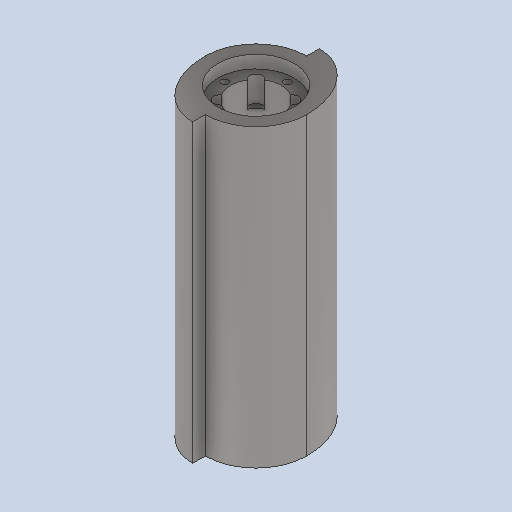
# Autodesk Inventor part: Деталь1
Saved by Autodesk Inventor 2024.2 (Build 282272000, 272)
## iProperties
Created: 2025-03-01
Part Number: Деталь1
Material: Сталь, литейная
Document SubType Name: Modeling
Designer: Timofey
Density: 7.85 g/cm^3
Appearance: С умеренной полировкой
Author: Timofey
Autodesk Inventor part; units mm, degrees
ref_plane "YZ Plane" through (0, 0, 0) normal (1, 0, 0) x (0, 1, 0)
ref_plane "XZ Plane" through (0, 0, 0) normal (0, 1, 0) x (-1, 0, 0)
ref_plane "XY Plane" through (0, 0, 0) normal (0, 0, 1) x (1, 0, 0)
sketch "Эскиз1" plane through (0, 0, 0) normal (0, 1, 0) x (-1, 0, 0)
  line L0 (0, 60) -> (0, 75)
  line L1 (0, -60) -> (0, -75)
  ellipse E0 centre (0, 0) end of major axis (0, -75) minor radius 60 (60, 0) -> (0, 75) ccw
  ellipse E1 centre (0, 0) end of major axis (0, -75) minor radius 60 (-60, 0) -> (0, -75) ccw
  arc A0 (0, 60) -> (-60, 0) centre (0, 0) ccw
  arc A1 (0, -60) -> (60, 0) centre (0, 0) ccw
  circle A2 centre (0, 0) radius 30
  dimension "d1" = 75
  dimension "d2" = 75
  dimension "d5" = 60
  constraints: 5 point on circle, 4 end point, 4 vertical, 3 centre point, 3 coincident, 9 other
  measures "d1" distance of A0.centre L0.end
  measures "d2" distance of A0.centre L1.end
  measures "d5" diameter of A2
extrude "Выдавливание1" add sketch "Эскиз1" along normal blind 350 contours L0 E0 A1 L1 E1 A0 | A2
sketch "Эскиз2" plane through (0, 0, 0) normal (0, -1, 0) x (1, 0, 0)
  ellipse E0 centre (0, 0) end of major axis (0, -75) minor radius 60 (0, 75) -> (-60, 0) ccw projected
  line L0 (0, 75) -> (0, 0)
  circle A0 centre (0, 0) radius 30
  line L1 (0, -75) -> (0, -60) projected
  line L2 (0, 0) -> (0, -75)
  line L3 (0, 0) -> (26.5165, -26.5165)
  line L4 (0, 0) -> (37.5, 0) construction
  line L5 (0, 0) -> (-26.5165, -26.5165)
  line L6 (0, 0) -> (37.5, 0) construction
  line L7 (0, 0) -> (-26.5165, 26.5165)
  line L8 (0, 0) -> (37.5, 0) construction
  line L9 (0, 0) -> (26.5165, 26.5165)
  line L10 (0, 0) -> (37.5, 0) construction
  circle A1 centre (26.5165, 26.5165) radius 5
  circle A2 centre (26.5165, -26.5165) radius 5
  circle A3 centre (-26.5165, 26.5165) radius 5
  circle A4 centre (-26.5165, -26.5165) radius 5
  circle A5 centre (0, 0) radius 45
  line L11 (0, 0) -> (30, 0)
  circle A6 centre (30, 0) radius 5
  line L12 (0, 0) -> (0, -30)
  circle A7 centre (0, -30) radius 5
  line L13 (0, 0) -> (-30, 0)
  circle A8 centre (-30, 0) radius 5
  line L14 (0, 0) -> (0, 30)
  circle A9 centre (0, 30) radius 5
  dimension "d13" = 60
  dimension "d14" = 37.5
  dimension "d15" = 45
  dimension "d16" = 37.5
  dimension "d17" = 135
  dimension "d18" = 37.5
  dimension "d19" = 135
  dimension "d20" = 37.5
  dimension "d21" = 45
  dimension "d22" = 10
  dimension "d23" = 10
  dimension "d24" = 10
  dimension "d25" = 10
  dimension "d26" = 90
  dimension "d30" = 30
  dimension "d31" = 30
  dimension "d32" = 30
  dimension "d33" = 30
  constraints: 28 end point, 10 centre point, 10 coincident, 5 horizontal, 4 equal length, 3 point on line, 1 collinear, 1 perpendicular, 1 vertical, 1 other
  measures "d13" diameter of A0
  measures "d14" distance of L2.start L3.end
  measures "d15" angle of L3 L4
  measures "d16" distance of L2.start L5.end
  measures "d17" angle of L5 L6
  measures "d18" distance of L2.start L7.end
  measures "d19" angle of L8 L7
  measures "d20" distance of L2.start L9.end
  measures "d21" angle of L10 L9
  measures "d22" diameter of A1
  measures "d23" diameter of A2
  measures "d24" diameter of A3
  measures "d25" diameter of A4
  measures "d26" diameter of A5
  measures "d30" distance of L11.start L11.end
  measures "d31" distance of L11.start L12.end
  measures "d32" distance of L11.start L13.end
  measures "d33" distance of L11.start L14.end
hole "Отверстие1" at (0, 0, 0) direction (0, 1, 0) diameter 60 end through all counterbore diameter 90 counterbore depth 15
sketch "Эскиз3" plane through (0, 0, 0) normal (0, -1, 0) x (1, 0, 0)
  line L0 (0, 0) -> (30, 0)
  circle A0 centre (30, 0) radius 5
  line L1 (0, 0) -> (0, -30)
  circle A1 centre (0, 0) radius 30 projected
  circle A2 centre (0, -30) radius 5
  line L2 (0, 0) -> (-30, 0)
  line L3 (0, 0) -> (0, 30)
  circle A3 centre (0, 30) radius 5
  circle A4 centre (-30, 0) radius 5
  dimension "d34" = 30
  dimension "d35" = 10
  dimension "d36" = 10
  dimension "d37" = 10
  dimension "d38" = 10
  constraints: 8 end point, 4 centre point, 4 coincident, 3 point on circle, 2 horizontal, 2 vertical
  measures "d34" distance of L0.start L0.end
  measures "d35" diameter of A0
  measures "d36" diameter of A2
  measures "d37" diameter of A3
  measures "d38" diameter of A4
hole "Отверстие2" at (0, 0, 30) at (-30, 0, 0) at (0, 0, -30) at (30, 0, 0) direction (0, 1, 0) diameter 15 depth 45
sketch "Эскиз5" plane through (0, 350, 0) normal (0, 1, 0) x (1, 0, 0)
  circle A0 centre (0, 0) radius 45
  constraints: 1 centre point, 1 coincident
hole "Отверстие4" at (0, 350, 0) direction (0, -1, 0) diameter 90 depth 15
sketch "Эскиз6" plane through (0, 335, 0) normal (0, 1, 0) x (1, 0, 0)
  line L0 (0, 0) -> (0, -37.5)
  line L1 (0, 0) -> (-37.5, 0)
  line L2 (0, 0) -> (0, 37.5)
  line L3 (0, 0) -> (37.5, 0)
  line L4 (0, 0) -> (-21.2132, -21.2132)
  line L5 (0, 0) -> (30, 0) construction
  line L6 (0, 0) -> (21.2132, -21.2132)
  line L7 (0, 0) -> (30, 0) construction
  line L8 (0, 0) -> (-21.2132, 21.2132)
  line L9 (0, 0) -> (30, 0) construction
  line L10 (0, 0) -> (21.2132, 21.2132)
  line L11 (0, 0) -> (30, 0) construction
  circle A0 centre (21.2132, -21.2132) radius 7.5
  circle A1 centre (-21.2132, -21.2132) radius 7.5
  circle A2 centre (-21.2132, 21.2132) radius 7.5
  circle A3 centre (21.2132, 21.2132) radius 7.5
  circle A4 centre (37.5, 0) radius 5
  circle A5 centre (0, -37.5) radius 5
  circle A6 centre (-37.5, 0) radius 5
  circle A7 centre (0, 37.5) radius 5
  dimension "d71" = 37.5
  dimension "d72" = 37.5
  dimension "d73" = 37.5
  dimension "d74" = 37.5
  dimension "d75" = 30
  dimension "d76" = 135
  dimension "d77" = 30
  dimension "d78" = 45
  dimension "d79" = 30
  dimension "d80" = 135
  dimension "d81" = 30
  dimension "d82" = 45
  dimension "d83" = 15
  dimension "d84" = 15
  dimension "d85" = 15
  dimension "d86" = 15
  dimension "d87" = 10
  dimension "d88" = 10
  dimension "d89" = 10
  dimension "d90" = 10
  constraints: 24 end point, 8 centre point, 8 coincident, 6 horizontal, 4 equal length, 2 vertical
  measures "d71" distance of L0.start L0.end
  measures "d72" distance of L0.start L1.end
  measures "d73" distance of L0.start L2.end
  measures "d74" distance of L0.start L3.end
  measures "d75" distance of L0.start L4.end
  measures "d76" angle of L4 L5
  measures "d77" distance of L0.start L6.end
  measures "d78" angle of L6 L7
  measures "d79" distance of L0.start L8.end
  measures "d80" angle of L9 L8
  measures "d81" distance of L0.start L10.end
  measures "d82" angle of L11 L10
  measures "d83" diameter of A0
  measures "d84" diameter of A1
  measures "d85" diameter of A2
  measures "d86" diameter of A3
  measures "d87" diameter of A4
  measures "d88" diameter of A5
  measures "d89" diameter of A6
  measures "d90" diameter of A7
hole "Отверстие5" at (21.2132, 335, 21.2132) at (-21.2132, 335, 21.2132) at (-21.2132, 335, -21.2132) at (21.2132, 335, -21.2132) direction (0, -1, 0) diameter 15 depth 30
sketch "Эскиз8" plane through (0, 335, 0) normal (0, 1, 0) x (1, 0, 0)
  point P0 (37, 0)
  point P1 (0, -37)
  point P2 (-37, 0)
  point P3 (0, 37)
hole "Отверстие7" at (37, 335, 0) at (0, 335, 37) at (-37, 335, 0) at (0, 335, -37) direction (0, -1, 0) diameter 8.376 depth 8 tip angle 120 thread size "M10x1.5" class "6H" standard "ISO Metric profile"
sketch "Эскиз9" plane through (0, 15, 0) normal (0, -1, 0) x (1, 0, 0)
  point P0 (26.163, 26.163)
  point P1 (26.163, -26.163)
  point P2 (-26.163, -26.163)
  point P3 (-26.163, 26.163)
hole "Отверстие8" at (26.163, 15, 26.163) at (26.163, 15, -26.163) at (-26.163, 15, -26.163) at (-26.163, 15, 26.163) direction (0, 1, 0) diameter 8.376 depth 8 tip angle 120 thread size "M10x1.5" class "6H" standard "ISO Metric profile"
